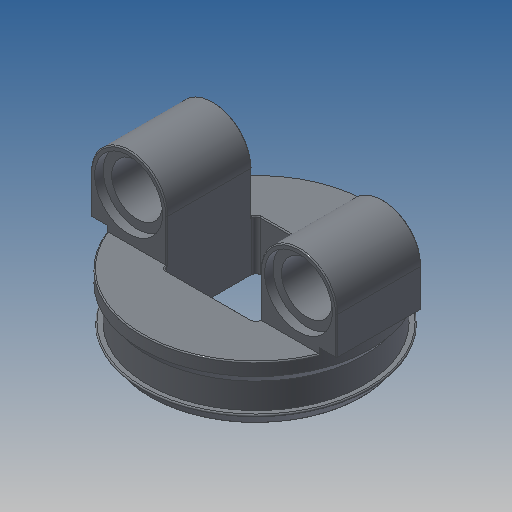
# Autodesk Inventor part: 99009-LtBluishGray
Saved by Autodesk Inventor 2022.2 (Build 262287000, 287)
## iProperties
Created: 2015-01-07
Part Number: 99009-LtBluishGray
Material: ABS Plastic
Document SubType Name: Modeling
Designer: D. Kohfeld
Density: 1.06 g/cm^3
Appearance: LtBluishGray
Mass: 1.3273 g
Surface Area: 21.2457 cm^2
Volume: 1.25217 cm^3
Author: D. Kohfeld
Autodesk Inventor part; units mm, degrees
ref_plane "YZ Plane" through (0, 0, 0) normal (1, 0, 0) x (0, 1, 0)
ref_plane "XZ Plane" through (0, 0, 0) normal (0, 1, 0) x (-1, 0, 0)
sketch "Sketch2" plane through (0, 0, 0) normal (1, 0, 0) x (0, 1, 0)
  line L0 (0, -9.24) -> (4, -9.24)
  line L1 (4, -9.24) -> (4, 0)
  line L2 (4, 0) -> (5.6, 0)
  line L3 (5.6, 0) -> (5.6, -10.8)
  line L4 (5.6, -10.8) -> (4.4, -10.8)
  line L5 (4.4, -10.8) -> (3.6, -10.2)
  line L6 (3.6, -10.2) -> (1.2, -10.2)
  line L7 (1.2, -10.8) -> (0, -9.9)
  line L8 (0, -9.9) -> (0, -9.24)
  line L9 (1.2, -10.8) -> (1.2, -10.2)
  point P0 (0, 0)
  dimension "d0" = 21.6
  dimension "d1" = 18.48
  dimension "d2" = 19.8
  dimension "d3" = 21.6
  dimension "d4" = 1.2
  dimension "d5" = 2.4
  dimension "d6" = 0.6
  dimension "d7" = 1.2
  dimension "d8" = 5.6
  dimension "d9" = 4
  constraints: 20 end point, 6 parallel, 1 horizontal, 1 horizontal alignment, 1 perpendicular, 1 vertical alignment
  measures "d0" diameter of L4 L2
  measures "d1" diameter of L0 L2
  measures "d2" diameter of L7.end L2
  measures "d3" diameter of L7.start L2
  measures "d4" distance between parallel lines of L9 L8
  measures "d5" distance from line of L5.end L9
  measures "d6" distance from line of L7.start L6
  measures "d7" distance from line of L4.end L3
  measures "d8" distance between parallel lines of L8 L3
  measures "d9" distance between parallel lines of L8 L1
revolve "Revolution1" add sketch "Sketch2" angle 360 about axis through (0, 4, 0) along (0, 1, 0)
ref_plane "Work Plane1" through (0, 0.8, 0) normal (0, -1, 0) x (1, 0, 0)
sketch "Sketch3" plane through (0, 0.8, 0) normal (0, -1, 0) x (1, 0, 0)
  line L0 (-4.4, 4) -> (-4.4, -4)
  arc A0 (-4.4, -4) -> (-4, -4.4) centre (-4, -4) ccw
  line L1 (-4, -4.4) -> (4, -4.4)
  arc A1 (4, -4.4) -> (4.4, -4) centre (4, -4) ccw
  line L2 (4.4, -4) -> (4.4, 4)
  arc A2 (4.4, 4) -> (4, 4.4) centre (4, 4) ccw
  line L3 (4, 4.4) -> (-4, 4.4)
  arc A3 (-4, 4.4) -> (-4.4, 4) centre (-4, 4) ccw
  line L4 (-4, 5.6) -> (4, 5.6)
  arc A4 (5.6, 4) -> (4, 5.6) centre (4, 4) ccw
  line L5 (5.6, 4) -> (5.6, -4)
  arc A5 (4, -5.6) -> (5.6, -4) centre (4, -4) ccw
  line L6 (4, -5.6) -> (-4, -5.6)
  arc A6 (-5.6, -4) -> (-4, -5.6) centre (-4, -4) ccw
  line L7 (-5.6, -4) -> (-5.6, 4)
  arc A7 (-4, 5.6) -> (-5.6, 4) centre (-4, 4) ccw
  point P0 (0, 0)
  point P1 (0, 4.4)
  point P2 (-4.4, 0)
  dimension "d12" = 0.4
  dimension "d13" = 8.8
  dimension "d14" = 1.2
  constraints: 16 end point, 16 point on circle, 8 centre point, 8 tangent, 4 parallel, 3 equal radius, 3 perpendicular, 2 midpoint, 1 horizontal alignment, 1 vertical, 1 vertical alignment, 7 other
  measures "d12" radius of A3
  measures "d13" distance between parallel lines of L1 L3
  measures "d14" distance between parallel lines of L3 L4
extrude "Extrusion1" add sketch "Sketch3" against normal up to next
extrude "Extrusion2" cut sketch "Sketch3" against normal through all contours A3 L3 A2 L2 A1 L1 A0 L0
sketch "Sketch4" plane through (0, 0, 0) normal (0, 0, 1) x (1, 0, 0)
  line L0 (-10.8, 5.6) -> (10.8, 5.6) projected
  circle A0 centre (-8, 9.6) radius 2.4
  circle A1 centre (8, 9.6) radius 2.4
  line L1 (4.4, 6) -> (4.4, 9.6)
  arc A2 (11.6, 9.6) -> (4.4, 9.6) centre (8, 9.6) ccw
  line L2 (11.6, 9.6) -> (11.6, 6)
  line L3 (11.6, 6) -> (4.4, 6)
  line L4 (-4.4, 6) -> (-4.4, 9.6)
  arc A3 (-4.4, 9.6) -> (-11.6, 9.6) centre (-8, 9.6) ccw
  line L5 (-11.6, 9.6) -> (-11.6, 6)
  line L6 (-11.6, 6) -> (-4.4, 6)
  line L7 (-4.4, 6) -> (4.4, 6) construction
  line L8 (0, 6) -> (0, 5.6) construction
  point P0 (0, 0)
  dimension "d19" = 4.8
  dimension "d20" = 7.2
  dimension "d21" = 16
  dimension "d22" = 4
  dimension "d23" = 0.4
  constraints: 16 end point, 4 centre point, 4 point on circle, 4 tangent, 2 concentric, 2 equal radius, 2 midpoint, 2 parallel, 1 horizontal alignment, 1 perpendicular, 1 vertical, 4 other
  measures "d19" diameter of A1
  measures "d20" diameter of A2
  measures "d21" distance of A0.centre A1.centre
  measures "d22" distance from line of A1.centre L0
extrude "Extrusion3" add sketch "Sketch4" along normal mid plane 8
sketch "Sketch5" plane through (0, 5.6, 0) normal (0, 1, 0) x (1, 0, 0)
  line L0 (4.4, 4) -> (4.4, -4)
  line L1 (-4.4, -4) -> (-4.4, 4)
  circle A0 centre (0, 0) radius 10.8
  line L2 (4.4, -4) -> (11.6, -4)
  line L3 (11.6, 4) -> (4.4, 4)
  line L4 (-4.4, 4) -> (-11.6, 4)
  line L5 (-11.6, -4) -> (-4.4, -4)
  line L6 (-4.4, 4) -> (-10.031949, 4)
  line L7 (-4.4, -4) -> (-10.031949, -4)
  line L8 (4.4, -4) -> (10.031949, -4)
  line L9 (4.4, 4) -> (10.031949, 4)
  constraints: 8 end point, 4 point on circle, 4 point on line
extrude "Extrusion4" add sketch "Sketch5" along normal up to next contours L3 A0 L2 L0 | L4 L1 L5 A0
sketch "Sketch6" plane through (0, 4, 0) normal (0, -1, 0) x (1, 0, 0)
  circle A0 centre (0, 0) radius 9.24
  line L0 (5.6, 4) -> (5.6, -4)
  line L1 (-5.6, -4) -> (-5.6, 4)
  line L2 (5.6, 2.3915) -> (8.925151, 2.3915)
  line L3 (5.6, -2.3915) -> (8.925151, -2.3915)
  line L4 (-5.6, 2.3915) -> (-8.925151, 2.3915)
  line L5 (-5.6, -2.3915) -> (-8.925151, -2.3915)
  dimension "d28" = 4.783
  constraints: 8 end point, 6 parallel, 4 point on circle, 4 point on line, 1 perpendicular
  measures "d28" distance between parallel lines of L2 L3
extrude "Extrusion5" cut sketch "Sketch6" against normal blind 1.6 contours A0 L3 L0 L2 | L4 L1 L5 A0
sketch "Sketch7" plane through (0, 0, 4) normal (0, 0, 1) x (1, 0, 0)
  circle A0 centre (8, 9.6) radius 2.4
  arc A1 (-4.4, 9.6) -> (-11.6, 9.6) centre (-8, 9.6) ccw
  line L0 (-4.4, 9.6) -> (-4.4, 5.6)
  line L1 (-10.031949, 5.6) -> (-4.4, 5.6)
  line L2 (-10.031949, 5.6) -> (-10.031949, 6)
  line L3 (-10.031949, 6) -> (-11.6, 6)
  line L4 (-11.6, 6) -> (-11.6, 9.6)
  circle A2 centre (-8, 9.6) radius 2.4
  circle A3 centre (-8, 9.6) radius 3.2
  circle A4 centre (8, 9.6) radius 3.2
  point P0 (0, 0)
  dimension "d31" = 6.4
  constraints: 2 centre point, 2 coincident, 1 equal radius
  measures "d31" diameter of A4
extrude "Extrusion6" cut sketch "Sketch7" against normal blind 0.8 contours A3 | A4
mirror "Mirror1" about plane through (0, 0, 0) normal (0, 0, 1) of "Extrusion6"
fillet "Fillet1" radius 0.1 48 edges at (-11.6, 7.8, 4) (-4.4, 7.6, 4) (-8, 13.2, 4) (-4.4, 7.6, -4) (-11.6, 7.8, -4) (-8, 13.2, -4) (4.2828, 5.6, -4.2828) (-4.2828, 5.6, -4.2828) (0, 5.6, -4.4) (-4.2828, 5.6, 4.2828) (4.2828, 5.6, 4.2828) (0, 5.6, 4.4) (4.4, 7.6, 4) (11.6, 7.8, 4) (8, 13.2, 4) (11.6, 7.8, -4) (4.4, 7.6, -4) (8, 13.2, -4) (11.6, 6, 0) (10.816, 6, 4) (10.0319, 5.8, 4) (10.816, 6, -4) (10.0319, 5.8, -4) (-10.816, 6, 4) (-10.0319, 5.8, 4) (-10.816, 6, -4) (0, 5.6, 10.8) (-6.0597, 5.6, -8.9398) (6.0597, 5.6, -8.9398) (-10.0319, 5.8, -4) (0, 0, 9.9) (0, 1.2, 10.8) (5.1314, 0.8, -5.1314) (0, 0.8, -5.6) (-5.1314, 0.8, -5.1314) (-5.6, 0.8, 0) (-5.1314, 0.8, 5.1314) (0, 0.8, 5.6) (5.1314, 0.8, 5.1314) (5.6, 0.8, 0) (4.2828, 0.8, -4.2828) (0, 0.8, -4.4) (-4.2828, 0.8, -4.2828) (-4.4, 0.8, 0) (-4.2828, 0.8, 4.2828) (0, 0.8, 4.4) (4.2828, 0.8, 4.2828) (4.4, 0.8, 0)
equation "\"d19\" = tpd"
equation "\"d20\" = tlad"
equation "\"d21\" = 2 * lu"
equation "\"d22\" = 0.5 * lu"
equation "\"d24\" = lu"
equation "\"d26\" = lu"
equation "\"d29\" = wall"
equation "\"d31\" = tsd"
equation "\"d32\" = tsl"
equation "\"tpd\" = 4.8"
equation "\"tlad\" = 7.2"
equation "\"lu\" = 8"
equation "\"wall\" = 1.6"
equation "\"tsd\" = 6.4"
equation "\"tsl\" = 0.8"
body "Solid1"
